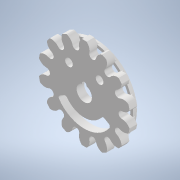
# Autodesk Inventor part: EnclosureFace
Saved by Autodesk Inventor 2020 (Build 240168000, 168)
## iProperties
Created: 2020-10-17
Part Number: EnclosureFace
Material: Generic
Document SubType Name: Modeling
Designer: vmiguel
Density: 1 g/cm^3
Appearance: Default
Author: vmiguel
Autodesk Inventor part; units mm, degrees
ref_plane "YZ Plane" through (0, 0, 0) normal (1, 0, 0) x (0, 1, 0)
ref_plane "XZ Plane" through (0, 0, 0) normal (0, 1, 0) x (-1, 0, 0)
ref_plane "XY Plane" through (0, 0, 0) normal (0, 0, 1) x (1, 0, 0)
sketch "Sketch1" plane through (0, 0, 0) normal (0, 0, 1) x (1, 0, 0)
  circle A0 centre (0, 0) radius 53.7665
  circle A1 centre (0, 0) radius 50.1
  dimension "d0" = 100.2
  constraints: 2 centre point, 2 coincident
  measures "d0" diameter of A1
extrude "Extrusion1" add sketch "Sketch1" against normal blind 5
sketch "Sketch2" plane through (0, 0, 0) normal (0, 0, 1) x (1, 0, 0)
  circle A0 centre (0, 0) radius 60
  dimension "d3" = 120
  constraints: 1 centre point, 1 coincident
  measures "d3" diameter of A0
extrude "Extrusion2" add sketch "Sketch2" along normal blind 10
sketch "Sketch3" plane through (0, 0, 10) normal (0, 0, 1) x (1, 0, 0)
  circle A0 centre (0, 0) radius 10
  circle A1 centre (0, 10) radius 3
  point P0 (2.9661, 9.55)
  point P1 (-2.9661, 9.55)
  dimension "d6" = 20
  dimension "d7" = 6
  constraints: 1 centre point, 1 coincident, 1 vertical alignment, 3 other
  measures "d7" diameter of A1
extrude "Extrusion3" cut sketch "Sketch3" against normal blind 10
sketch "Sketch4" plane through (0, 0, 10) normal (0, 0, 1) x (1, 0, 0)
  arc A0 (-22.3478, -16.0259) -> (22.3478, -16.0259) centre (0, 0) ccw
  arc A1 (-32.9053, -22.7429) -> (32.9053, -22.7429) centre (0, 0) ccw
  line L0 (-26.2857, -15.1761) -> (-31.9374, -18.4391)
  line L1 (26.2857, -15.1761) -> (31.9374, -18.4391)
  line L2 (0, 84) -> (0, -84) projected
  arc A2 (-31.9374, -18.4391) -> (-32.9053, -22.7429) centre (-30.4374, -21.0372) ccw
  arc A3 (32.9053, -22.7429) -> (31.9374, -18.4391) centre (30.4374, -21.0372) ccw
  arc A4 (26.2857, -15.1761) -> (22.3478, -16.0259) centre (24.7857, -17.7741) ccw
  arc A5 (-22.3478, -16.0259) -> (-26.2857, -15.1761) centre (-24.7857, -17.7741) ccw
  point P0 (34.641, -20)
  point P1 (-34.641, -20)
  point P2 (23.8157, -13.75)
  point P3 (-23.8157, -13.75)
  dimension "d10" = 55
  dimension "d11" = 80
  dimension "d12" = 120
  dimension "d13" = 60
  dimension "d14" = 3
  constraints: 16 point on circle, 8 tangent, 6 centre point, 6 point on line, 4 end point, 3 equal radius, 2 coincident
  measures "d10" diameter of A0
  measures "d11" diameter of A1
  measures "d12" angle of L1 L0
  measures "d13" angle of L1 L2
  measures "d14" radius of A2
extrude "Extrusion4" cut sketch "Sketch4" against normal blind 10
sketch "Sketch5" plane through (0, 0, 10) normal (0, 0, 1) x (1, 0, 0)
  circle A0 centre (-20, 25) radius 5
  circle A1 centre (20, 25) radius 5
  point P0 (0, 0)
  dimension "d17" = 20
  dimension "d18" = 20
  dimension "d19" = 25
  dimension "d20" = 10
  constraints: 2 centre point, 1 equal radius, 1 horizontal alignment
  measures "d17" horizontal distance of A0.centre point (0, 0)
  measures "d18" horizontal distance of A1.centre point (0, 0)
  measures "d19" vertical distance of A1.centre point (0, 0)
  measures "d20" diameter of A1
extrude "Extrusion5" cut sketch "Sketch5" against normal blind 10
sketch "Sketch6" plane through (0, 0, 10) normal (0, 0, 1) x (1, 0, 0)
  circle A0 centre (0, 0) radius 60 projected
  line L0 (0, 0) -> (26.033, 54.0581)
  line L1 (0, 84) -> (0, -84) projected
  arc A1 (3.1402, 59.9178) -> (0, 60) centre (0, 0) ccw
  arc A2 (26.033, 54.0581) -> (23.1682, 55.3465) centre (0, 0) ccw
  line L2 (3.1402, 59.9178) -> (0, 0)
  line L3 (23.1682, 55.3465) -> (0, 0)
  arc A3 (6.6548, 49.0098) -> (15.2688, 47.0437) centre (10.9618, 48.0268) ccw
  line L4 (2.6168, 49.9315) -> (19.3068, 46.1221) construction
  arc A4 (6.6548, 49.0098) -> (3.1402, 59.9178) centre (-4.2819, 51.5061) ccw
  arc A5 (23.1682, 55.3465) -> (15.2688, 47.0437) centre (26.2055, 44.5475) ccw
  dimension "d23" = 25.714
  dimension "d24" = 3
  dimension "d25" = 3
  dimension "d28" = 10
  dimension "d29" = 10
  constraints: 15 point on circle, 8 end point, 5 centre point, 5 point on line, 2 equal radius, 2 midpoint, 2 tangent, 1 coincident, 1 concentric
  measures "d23" angle of L0 L1
  measures "d24" angle of L1 L2
  measures "d25" angle of L0 L3
  measures "d28" distance of L3.start L4.end
  measures "d29" distance of L4.start L2.start
extrude "Extrusion6" cut sketch "Sketch6" against normal blind 10 contours A5 A3 A4 A0
pattern_circular "Circular Pattern1" count 14 over 360 about axis through (0, 0, 0) along (0, 0, 1) of "Extrusion6"
fillet "Fillet1" radius 4 14 edges at (0, 53.7665, 0) (-23.3284, 48.4419, 0) (-42.0363, 33.5229, 0) (23.3284, 48.4419, 0) (42.0363, 33.5229, 0) (-52.4185, 11.9642, 0) (-52.4185, -11.9642, 0) (-42.0363, -33.5229, 0) (-23.3284, -48.4419, 0) (0, -53.7665, 0) (23.3284, -48.4419, 0) (42.0363, -33.5229, 0) (52.4185, -11.9642, 0) (52.4185, 11.9642, 0)
equation "\"d13\" = 0.5 * d12"
equation "\"d18\" = d17"
equation "\"d25\" = d24"
equation "\"d29\" = d28"
body "Solid1"
